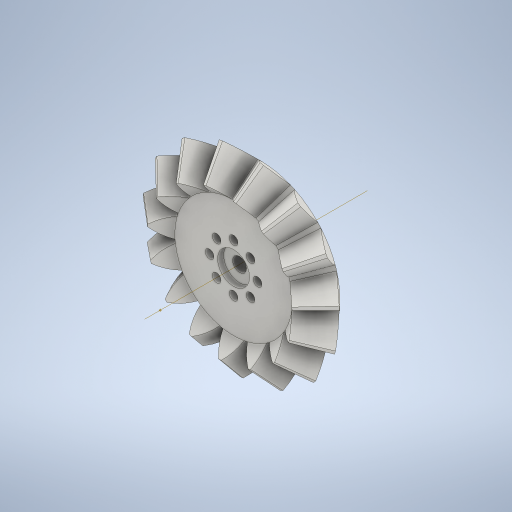
# Autodesk Inventor part: かさ歯車1
Saved by Autodesk Inventor 2024 (Build 280153000, 153)
## iProperties
CustomPartVersion: 1
Created: 2024-07-09
Part Number: かさ歯車1
Material: Steel, Mild
Document SubType Name: Modeling
Designer: right
Categories: <?xml version="1.0" encoding="UTF-16"?> <MemberInstance><Categories><FamilyTemplate><FamilyTemplateParameter ValueType="xs:double" Id="1" ObjectReferenceKey="da_z" ObjectType="kUserParameterObject"/><FamilyTemplateParameter ValueType="xs:double" Id="2" ObjectReferenceKey="da_b" ObjectType="kUserParameterObject"/><FamilyTemplateParameter ValueType="xs:double" Id="3" ObjectReferenceKey="da_beta" ObjectType="kUserParameterObject"/><FamilyTemplateParameter ValueType="xs:double" Id="4" ObjectReferenceKey="da_dae" ObjectType="kUserParameterObject"/><FamilyTemplateParameter ValueType="xs:double" Id="5" ObjectReferenceKey="da_ve" ObjectType="kUserParameterObject"/><FamilyTemplateParameter ValueType="xs:double" Id="6" ObjectReferenceKey="da_omega" ObjectType="kUserParameterObject"/><FamilyTemplateParameter ValueType="xs:string" Id="7" ObjectReferenceKey="EAIAABAAAAAAHwAAAAAAAIAAAAAAAAAA" ObjectType="83914240" SubObjectId="SurfaceGeometry"/></FamilyTemplate><ParamToTemplateMap><ParamToTemplate CategoryParameter="//CategoryParameter[@InternalName='046C89C9-8512-4d59-83FE-43B91F4F132A']" TemplateParameter="1"/><ParamToTemplate CategoryParameter="//CategoryParameter[@InternalName='2552DF32-E462-4b46-AEBF-C6C7768E72AC']" TemplateParameter="2"/><ParamToTemplate CategoryParameter="//CategoryParameter[@InternalName='C9EE641D-15FC-4fae-A226-E94C4372FDD7']" TemplateParameter="3"/><ParamToTemplate><ParamToTemplate CategoryParameter="//CategoryParameter[@InternalName='00B6519A-459B-49c7-AD84-2E56D39A5744']" ConstantValue="0.000000"/></ParamToTemplate><ParamToTemplate><ParamToTemplate CategoryParameter="//CategoryParameter[@InternalName='04B31F0E-C7A6-4894-AA32-9629BEFACF47']" ConstantValue="1.000000"/></ParamToTemplate><ParamToTemplate><ParamToTemplate CategoryParameter="//CategoryParameter[@InternalName='43CBEC2E-7847-49e7-A936-2F7889FCB2D9']" ConstantValue="0.200000"/></ParamToTemplate><ParamToTemplate><ParamToTemplate CategoryParameter="//CategoryParameter[@InternalName='B1EFC894-105D-4ebd-86BF-FA20ED196853']" ConstantValue="0.300000"/></ParamToTemplate><ParamToTemplate><ParamToTemplate CategoryParameter="//CategoryParameter[@InternalName='51175063-3D10-4879-93E8-6246FE8B403D']" ConstantValue="2060000000.000000"/></ParamToTemplate><ParamToTemplate><ParamToTemplate CategoryParameter="//CategoryParameter[@InternalName='A3A52E27-4454-46a9-B0BD-C932399B70AF']" ConstantValue="0.300000"/></ParamToTemplate><ParamToTemplate CategoryParameter="//CategoryParameter[@InternalName='2A200944-5A8C-41ca-B96E-8520D2E510F1']" TemplateParameter="4"/><ParamToTemplate><ParamToTemplate CategoryParameter="//CategoryParameter[@InternalName='1A637F62-92C8-44bc-B81F-10802510B579']" ConstantValue="3.624325"/></ParamToTemplate><ParamToTemplate CategoryParameter="//CategoryParameter[@InternalName='B52DD4BE-6863-48fb-BF58-89EF6F9EC65C']" TemplateParameter="5"/><ParamToTemplate><ParamToTemplate CategoryParameter="//CategoryParameter[@InternalName='3956BFF2-84D2-457d-93C2-9B0613DEBA67']" ConstantValue="1.499898"/></ParamToTemplate><ParamToTemplate CategoryParameter="//CategoryParameter[@InternalName='739CFA02-461B-4bf8-8049-181FCAD8B28F']" TemplateParameter="6"/><ParamToTemplate><ParamToTemplate CategoryParameter="//CategoryParameter[@InternalName='A27E999F-E2CE-4481-8A2A-EBF499C4C3C5']" ConstantValue="0.000000"/></ParamToTemplate><ParamToTemplate><ParamToTemplate CategoryParameter="//CategoryParameter[@InternalName='9E1B4470-B2D3-4ff1-B813-535BB4CDF51A']" ConstantValue="3520000.000000"/></ParamToTemplate><ParamToTemplate><ParamToTemplate CategoryParameter="//CategoryParameter[@InternalName='F8452263-BFF6-458c-9FB1-07C4B99E95CD']" ConstantValue="11400000.000000"/></ParamToTemplate><ParamToTemplate><ParamToTemplate CategoryParameter="//CategoryParameter[@InternalName='3E3BB259-FD49-497f-8171-6EBC954A3479']" ConstantValue="2.000000"/></ParamToTemplate><ParamToTemplate CategoryParameter="//CategoryParameter[@InternalName='27C3BAF2-7550-4e4b-AE2C-0DB134B7D9B7']" TemplateParameter="7"/></ParamToTemplateMap><Category DisplayName="Gear" InternalName="DC85795E-93AB-48d5-8EEE-5A27447B64BD" Mnemonic="Gear"><CategoryParameter DisplayName="z" InternalName="046C89C9-8512-4d59-83FE-43B91F4F132A" Mnemonic="z"/><CategoryParameter DisplayName="b" InternalName="2552DF32-E462-4b46-AEBF-C6C7768E72AC" Mnemonic="b"/><CategoryParameter DisplayName="||b|" InternalName="C9EE641D-15FC-4fae-A226-E94C4372FDD7" Mnemonic="beta"/><CategoryParameter DisplayName="x" InternalName="00B6519A-459B-49c7-AD84-2E56D39A5744" Mnemonic="x"/><CategoryParameter DisplayName="a*" InternalName="04B31F0E-C7A6-4894-AA32-9629BEFACF47" Mnemonic="a"/><CategoryParameter DisplayName="c*" InternalName="43CBEC2E-7847-49e7-A936-2F7889FCB2D9" Mnemonic="c"/><CategoryParameter DisplayName="r|.f|*" InternalName="B1EFC894-105D-4ebd-86BF-FA20ED196853" Mnemonic="rf"/><CategoryParameter DisplayName="E" InternalName="51175063-3D10-4879-93E8-6246FE8B403D" Mnemonic="E"/><CategoryParameter DisplayName="||m|" InternalName="A3A52E27-4454-46a9-B0BD-C932399B70AF" Mnemonic="mi"/><Category DisplayName="BevelGear" InternalName="0C98F69A-0C2B-4791-B2FE-7691BB227E77" Mnemonic="BevelGear"><CategoryParameter DisplayName="d|.ae|" InternalName="2A200944-5A8C-41ca-B96E-8520D2E510F1" Mnemonic="dae"/><CategoryParameter DisplayName="d|.ai|" InternalName="1A637F62-92C8-44bc-B81F-10802510B579" Mnemonic="dai"/><CategoryParameter DisplayName="J|.e|" InternalName="B52DD4BE-6863-48fb-BF58-89EF6F9EC65C" Mnemonic="ve"/><CategoryParameter DisplayName="J|.i|" InternalName="3956BFF2-84D2-457d-93C2-9B0613DEBA67" Mnemonic="vi"/><CategoryParameter DisplayName="||S|" InternalName="739CFA02-461B-4bf8-8049-181FCAD8B28F" Mnemonic="omega"/><CategoryParameter DisplayName="x|.t|" InternalName="A27E999F-E2CE-4481-8A2A-EBF499C4C3C5" Mnemonic="xt"/><CategoryParameter DisplayName="||s||.Flim|" InternalName="9E1B4470-B2D3-4ff1-B813-535BB4CDF51A" Mnemonic="sFlim"/><CategoryParameter DisplayName="||s||.Hlim|" InternalName="F8452263-BFF6-458c-9FB1-07C4B99E95CD" Mnemonic="sHlim"/><CategoryParameter DisplayName="タイプ" InternalName="3E3BB259-FD49-497f-8171-6EBC954A3479" Mnemonic="type"/><CategoryParameter DisplayName="PitchDiameter" InternalName="27C3BAF2-7550-4e4b-AE2C-0DB134B7D9B7" Mnemonic="IDS_PITCHDIAM"/></Category></Category></Categories></MemberInstance>
Mass: 60.9118 g
Surface Area: 34.3074 cm^2
Volume: 7.7496 cm^3
Density: 7.86 g/cm^3
Appearance: Steel
Author: right
Autodesk Inventor part; units mm, degrees
ref_plane "メッシュ平面2" through (0, 0, 0) normal (0.9781476, 0.2079117, 0) x (0, 0, 1)
sketch "歯のボディ スケッチ" plane through (0, 0, 0) normal (1, 0, 0) x (0, 1, 0)
  line L0 (0, 0) -> (19.954416, -25.045584) construction
  line L1 (19.954416, -25.045584) -> (24.62132, -20.37868)
  line L2 (24.62132, -20.37868) -> (0, 0) construction
  line L3 (22.5, -22.5) -> (0, 0) construction
  line L4 (14.686719, -18.433887) -> (18.121623, -14.998983)
  line L5 (19.954416, -25.045584) -> (14.686719, -18.433887)
  line L6 (24.62132, -20.37868) -> (18.121623, -14.998983)
  line L7 (0, -39.386751) -> (0, 6.564458)
  line L8 (0, -22.5) -> (24.62132, -22.5) construction
  dimension "d0" = 45
  dimension "d1" = 39.90883
  dimension "d2" = 49.24264
  dimension "d3" = 8.4
  dimension "d4" = 20.37868
  constraints: 16 end point, 4 point on line, 3 perpendicular, 2 collinear, 1 horizontal alignment, 1 vertical alignment
  measures "d0" diameter of L3.start L7
  measures "d1" diameter of L0.end L7
  measures "d2" diameter of L1.end L7
  measures "d3" distance between parallel lines of L1 L4
  measures "d4" vertical distance of L1.end L0.start
revolve "歯のボディ" add sketch "歯のボディ スケッチ" angle 360 about axis through (0, 0, 0) along (0, 0, 1)
ref_plane "歯の平面" through (0, 22.5, -22.5) normal (0, -0.7071068, 0.7071068) x (1, 0, 0)
sketch "開始スケッチ" plane through (0, 22.5, -22.5) normal (0, -0.7071068, 0.7071068) x (1, 0, 0)
  line L0 (0, -23.505131) -> (0, 10.644758)
  arc A0 (-0.31611, -4.392) -> (-6.776444, 4.350701) centre (-16.176375, -9.353538) ccw
  arc A1 (6.776444, 4.350701) -> (0.31611, -4.392) centre (16.176375, -9.353538) ccw
  line L1 (-0.31611, -4.392) -> (0.31611, -4.392)
  arc A2 (6.776444, 4.350701) -> (-6.776444, 4.350701) centre (0, -31.819805) ccw
  dimension "d7" = 16.61821
  dimension "d8" = 16.17637
  dimension "d9" = 22.46627
  dimension "d57" = 36.79981
  dimension "d58" = 27.42781
  constraints: 6 point on circle, 3 centre point, 3 symmetric about line, 2 end point, 1 coincident, 1 perpendicular, 1 other
  measures "d7" radius of A0
  measures "d8" horizontal distance of point (0, -31.82) A0.centre
  measures "d9" vertical distance of point (0, -31.82) A0.centre
  measures "d57" radius of A2
  measures "d58" distance from line of A2.centre L1
ref_plane "終了平面" through (0, 16.326958, -16.326958) normal (0, -0.7071068, 0.7071068) x (1, 0, 0)
sketch "終了側スケッチ" plane through (0, 16.326958, -16.326958) normal (0, -0.7071068, 0.7071068) x (1, 0, 0)
  line L0 (0, -15.35404) -> (0, 6.953444)
  arc A0 (-0.229383, -3.187022) -> (-4.917277, 3.157053) centre (-11.738266, -6.787326) ccw
  arc A1 (4.917277, 3.157053) -> (0.229383, -3.187022) centre (11.738266, -6.787326) ccw
  line L1 (-0.229383, -3.187022) -> (0.229383, -3.187022)
  arc A2 (4.917277, 3.157053) -> (-4.917277, 3.157053) centre (0, -23.089805) ccw
  dimension "d12" = 12.05888
  dimension "d15" = 11.73827
  dimension "d16" = 16.30248
  dimension "d59" = 26.70351
  dimension "d60" = 19.90278
  constraints: 6 point on circle, 3 centre point, 3 symmetric about line, 2 end point, 1 coincident, 1 other
  measures "d12" radius of A0
  measures "d15" horizontal distance of A0.centre point (0, -23.09)
  measures "d16" vertical distance of A0.centre point (0, -23.09)
  measures "d59" radius of A2
  measures "d60" distance from line of A2.centre L1
loft "Loft" cut profiles "開始スケッチ", "終了側スケッチ"
pattern_circular "Circular Pattern" count 15 over 360 about axis through (0, 0, 0) along (0, 0, 1) of "Loft"
sketch3d "3D スケッチ(右)"
ref_plane "終了平面(右)" through (-2.644613, 16.111349, -16.326958) normal (0.114536, -0.697769, 0.7071068) x (0.9867943, 0.1619783, 0)
sketch "終了側スケッチ(右)" plane through (-2.644613, 16.111349, -16.326958) normal (0.114536, -0.697769, 0.7071068) x (0.9867943, 0.1619783, 0)
  arc A0 (-0.229383, -3.187022) -> (-4.917277, 3.157053) centre (-11.738266, -6.787326) ccw
  line L0 (0, -30.546139) -> (0, 11.222988)
  arc A1 (4.917277, 3.157053) -> (0.229383, -3.187022) centre (11.738266, -6.787326) ccw
  line L1 (-0.229383, -3.187022) -> (0.229383, -3.187022)
  arc A2 (4.917277, 3.157053) -> (-4.917277, 3.157053) centre (0, -23.089805) ccw
  dimension "d70" = 11.73827
  dimension "d71" = 16.30248
  dimension "d72" = 12.05888
  dimension "d73" = 19.90278
  dimension "d74" = 26.70351
  constraints: 6 point on circle, 3 centre point, 3 symmetric about line, 2 end point, 1 coincident, 1 perpendicular, 1 other
  measures "d70" horizontal distance of A2.centre A0.centre
  measures "d71" vertical distance of point (0, -23.09) A0.centre
  measures "d72" radius of A0
  measures "d73" distance from line of point (0, -23.09) L1
  measures "d74" radius of A2
feature "ロフト(右)" [suppressed]
pattern_circular "放射状パターン(右)" [suppressed]
sketch3d "3D スケッチ(左)"
ref_plane "終了平面(左)" through (2.672831, 16.111349, -16.339123) normal (-0.1156987, -0.697411, 0.7072706) x (0.9865167, -0.1636606, 0)
sketch "終了側スケッチ(左)" plane through (2.672831, 16.111349, -16.339123) normal (-0.1156987, -0.697411, 0.7072706) x (0.9865167, -0.1636606, 0)
  line L0 (0, -32.659382) -> (0, 13.343889)
  arc A0 (-0.229383, -3.181671) -> (-4.917277, 3.162405) centre (-11.738266, -6.781975) ccw
  arc A1 (4.917277, 3.162405) -> (0.229383, -3.181671) centre (11.738266, -6.781975) ccw
  line L1 (-0.229383, -3.181671) -> (0.229383, -3.181671)
  ellipse E0 centre (0, -10.603424) end of major axis (18.121623, -10.603424) minor radius 12.816892
  arc A2 (4.917277, 3.162405) -> (-4.917277, 3.162405) centre (0, -23.084454) ccw
  dimension "d56" = 12.81689
  dimension "d30" = 12.05888
  dimension "d31" = 11.73827
  dimension "d32" = 16.30248
  dimension "d61" = 26.70351
  dimension "d62" = 19.90278
  constraints: 6 point on circle, 3 centre point, 3 symmetric about line, 2 end point, 1 coincident, 2 other
  measures "d30" radius of A0
  measures "d31" horizontal distance of point (0, -23.084) A0.centre
  measures "d32" vertical distance of A0.centre point (0, -23.084)
  measures "d61" radius of A2
  measures "d62" distance from line of point (0, -23.084) L1
feature "ロフト(左)" [suppressed]
pattern_circular "放射状パターン(左)" [suppressed]
sketch "ボディ スケッチ" plane through (0, 0, 0) normal (1, 0, 0) x (0, 1, 0)
  line L0 (0, -35.037536) -> (0, -19.530831)
  line L1 (19.954416, -25.045584) -> (14.686719, -18.433887)
  line L2 (14.686719, -18.433887) -> (0, -18.433887)
  line L3 (19.954416, -25.045584) -> (0, -25.045584)
  constraints: 4 end point, 2 perpendicular, 2 point on line
sketch "ボディ スケッチ outline for 固定ボディ" plane through (0, 0, 0) normal (1, 0, 0) x (0, 1, 0)
  line L0 (0, -25.045584) -> (19.954416, -25.045584)
  line L1 (0, -18.433887) -> (0, -25.045584)
  line L2 (14.686719, -18.433887) -> (0, -18.433887)
  line L3 (19.954416, -25.045584) -> (14.686719, -18.433887)
revolve "固定ボディ" add sketch "ボディ スケッチ outline for 固定ボディ" angle 360 about axis through (0, 0, 0) along (0, 0, 1)
sketch "Sketch6" plane through (0, 0, 0) normal (1, 0, 0) x (0, 1, 0)
  line L0 (22.5, -22.5) -> (0, 0)
  line L1 (0, -37.799919) -> (0, 6.299986)
surface revolve "ピッチ円直径" sketch "Sketch6" angle 360 about axis through (0, 0, 0) along (0, 0, 1) shown no curves L0
sketch "スケッチ8" plane through (0, 0, -25.045584) normal (0, 0, -1) x (-1, 0, 0)
  circle A0 centre (0, 0) radius 4
  circle A1 centre (0, 0) radius 6 construction
  circle A2 centre (0, 6) radius 1.1
  circle A3 centre (-4.242641, 4.242641) radius 1.1
  circle A4 centre (-6, 0) radius 1.1
  circle A5 centre (-4.242641, -4.242641) radius 1.1
  circle A6 centre (0, -6) radius 1.1
  circle A7 centre (4.242641, -4.242641) radius 1.1
  circle A8 centre (6, 0) radius 1.1
  circle A9 centre (4.242641, 4.242641) radius 1.1
  dimension "d95" = 12
  dimension "d94" = 8
  dimension "d96" = 2.2
  dimension "d99" = 360
  constraints: 9 centre point, 2 coincident, 2 vertical alignment, 19 other
  measures "d94" diameter of A0
  measures "d96" diameter of A2
extrude "押し出し1" cut sketch "スケッチ8" against normal blind 10
sketch "スケッチ12" plane through (0, 0, -25.045584) normal (0, 0, -1) x (-1, 0, 0)
  circle A0 centre (0, 6) radius 1.1
  circle A1 centre (0, 6) radius 2
  circle A2 centre (0, 0) radius 4
  circle A3 centre (-4.242641, 4.242641) radius 2
  circle A4 centre (-6, 0) radius 2
  circle A5 centre (-4.242641, -4.242641) radius 2
  circle A6 centre (0, -6) radius 2
  circle A7 centre (4.242641, -4.242641) radius 2
  circle A8 centre (6, 0) radius 2
  circle A9 centre (4.242641, 4.242641) radius 2
  circle A10 centre (0, 0) radius 8
  dimension "d119" = 4
  dimension "d122" = 360
  constraints: 9 centre point, 2 coincident, 1 tangent, 17 other
  measures "d119" diameter of A1
extrude "押し出し6" cut sketch "スケッチ12" against normal blind 3 contours A0 | A1 | A1 A10 A9 A2 | A1 A2 A3 A10 | A2 | A10 A8 A2 A9 | A9 | A3 | A3 A2 A4 A10 | A8 | A10 A7 A2 A8 | A4 | A4 A2 A5 A10 | A10 A6 A2 A7 | A7 | A5 | A5 A2 A6 A10 | A6
sketch "スケッチ13" plane through (0, 0, -22.045584) normal (0, 0, -1) x (-1, 0, 0)
  circle A0 centre (0, 0) radius 4 projected
  circle A1 centre (0, 0) radius 3
  dimension "d126" = 6
  constraints: 1 centre point, 1 coincident
  measures "d126" diameter of A1
extrude "押し出し7" add sketch "スケッチ13" against normal blind 2.112
extrude "押し出し8" add sketch "スケッチ13" along normal up to surface (3 mm away)
fillet "フィレット2" radius 2 1 edges at (4, 0, -22.0456)
extrude "押し出し9" cut sketch "スケッチ12" against normal up to surface (3 mm away) contours A1 | A9 | A3 | A8 | A4 | A7 | A5 | A6
sketch "スケッチ14" plane through (0, 0, -19.933584) normal (0, 0, 1) x (1, 0, 0)
  circle A0 centre (0, 0) radius 3 projected
  circle A1 centre (0, 0) radius 1.75
  dimension "d134" = 3.5
  constraints: 1 centre point, 1 coincident
  measures "d134" diameter of A1
extrude "押し出し10" add sketch "スケッチ14" against normal blind 5
equation "\"d0\" = da_de"
equation "\"d1\" = da_dfe"
equation "\"d2\" = da_dae"
equation "\"d3\" = da_b"
equation "\"d4\" = da_ve"
equation "\"d7\" = fd_rr"
equation "\"d8\" = fd_x"
equation "\"d9\" = fd_y"
equation "\"d57\" = 0.5 * fd_dva + 0.3 * da_he"
equation "\"d58\" = 0.5 * fd_dva - 1.12 * da_he"
equation "\"da_teethtype\" = 0"
equation "\"da_b\" = 8.4"
equation "\"da_de\" = 45"
equation "\"da_dae\" = 49.24264"
equation "\"da_dfe\" = 39.90883"
equation "\"da_le\" = 31.81981"
equation "\"da_omega\" = 90deg"
equation "\"da_beta\" = 0"
equation "\"da_delta\" = 45deg"
equation "\"da_alpha\" = 30deg"
equation "\"da_he\" = 6.6"
equation "\"da_ve\" = 20.37868"
equation "\"da_zv\" = 21.213203"
equation "\"fd_loft\" = da_b + 0.05 * da_he"
equation "\"fd_x\" = fd_x1 + fd_x2"
equation "\"fd_y\" = fd_y1 - fd_y2"
equation "\"fd_dd\" = fd_dva - 0.8 * da_he"
equation "\"da_dvw\" = 63.63961"
equation "\"d11\" = fd_loft"
equation "\"da_dm\" = 39.0603"
equation "\"da_x\" = 0"
equation "\"da_m\" = 3"
equation "\"d50\" = da_omega"
equation "\"fd_rr\" = 16.618209"
equation "\"fd_dva\" = 69.63961"
equation "\"fd_x1\" = 2.380149"
equation "\"fd_x2\" = 13.796225"
equation "\"fd_y1\" = 31.730662"
equation "\"fd_y2\" = 9.264395"
body "Solid1"
body "Srf1"
